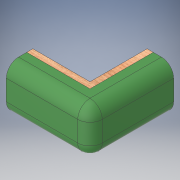
# Autodesk Inventor part: bumpers
Saved by Autodesk Inventor 2018 (Build 220112000, 112)
## iProperties
Created: 2019-04-28
Part Number: bumpers
Material: Generic
Document SubType Name: Modeling
Designer: corbin
Density: 1 g/cm^3
Appearance: Default
Author: corbin
Autodesk Inventor part; units mm, degrees
ref_plane "YZ Plane" through (0, 0, 0) normal (1, 0, 0) x (0, 1, 0)
ref_plane "XZ Plane" through (0, 0, 0) normal (0, 1, 0) x (-1, 0, 0)
ref_plane "XY Plane" through (0, 0, 0) normal (0, 0, 1) x (1, 0, 0)
sketch "Sketch1" plane through (0, 0, 0) normal (0, 1, 0) x (-1, 0, 0)
  line L0 (0, 0) -> (177.8, 0)
  line L1 (177.8, 0) -> (177.8, -19.05)
  line L2 (177.8, -19.05) -> (0, -19.05)
  line L3 (0, -19.05) -> (0, 0)
  line L4 (0, 0) -> (-19.05, 0)
  line L5 (-19.05, 0) -> (-19.05, -196.85)
  line L6 (-19.05, -196.85) -> (0, -196.85)
  line L7 (0, -196.85) -> (0, 0)
  dimension "d0" = 177.8
  dimension "d1" = 19.05
  dimension "d2" = 19.05
  dimension "d3" = 196.85
  constraints: 16 end point, 4 parallel, 2 horizontal, 2 perpendicular
  measures "d0" distance of L1.end L2.end
  measures "d1" distance of L0.end L1.end
  measures "d2" distance of L6.end L5.end
  measures "d3" distance of L5.end L4.end
extrude "Extrusion1" add sketch "Sketch1" along normal blind 139.7
sketch "Sketch3" plane through (0, 139.7, 0) normal (0, 1, 0) x (1, 0, 0)
  line L0 (19.05, 0) -> (19.05, 196.85) projected
  line L1 (19.05, 196.85) -> (82.55, 196.85)
  line L2 (82.55, 196.85) -> (82.55, 0)
  line L3 (19.05, 0) -> (19.05, 196.85)
  line L4 (-177.8, 0) -> (-177.8, -63.5)
  line L5 (-177.8, -63.5) -> (82.55, -63.5)
  line L6 (82.55, -63.5) -> (82.55, 0)
  line L7 (19.05, 196.85) -> (19.05, 0)
  line L8 (19.05, 0) -> (-177.8, 0)
  point P0 (0, 0)
  dimension "d11" = 63.5
  dimension "d12" = 260.35
  dimension "d13" = 63.5
  constraints: 16 end point, 3 parallel, 2 horizontal, 2 perpendicular, 1 vertical
  measures "d11" distance of L2.end L3.start
  measures "d12" distance of L5.end L4.end
  measures "d13" distance of L4.end L4.start
extrude "Extrusion3" add sketch "Sketch3" against normal blind 139.7 separate body
fillet "Fillet1" radius 38.1 5 edges at (-47.625, 0, 63.5) (82.55, 0, 31.75) (82.55, 69.85, 63.5) (-47.625, 139.7, 63.5) (82.55, 139.7, -98.425)
body "Solid1"
body "Solid2"
